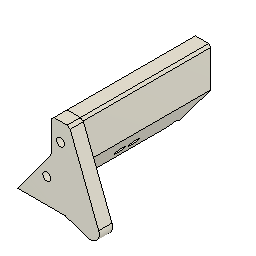
doctor-blade-coater (Autodesk Fusion 360 design; units mm, degrees)
Autodesk Fusion 360 part; units mm, degrees
note: some values were not read from the file. Set by a fixed rule: which sketch regions a step uses; the direction of a hole.
sketch "Blade Stock Layout and Angle setting" plane through (0, 0, 0) normal (0, 0, 1) x (1, 0, 0) in component "Blade"
  line L0 (0, 1.52) -> (0.9475, 3.3067)
  line L1 (0, 1.52) -> (1.43, 2.95)
  line L2 (0.9475, 3.3067) -> (1.43, 2.95) construction
  line L3 (1.43, 2.95) -> (11.5347, 16.621)
  line L4 (11.5347, 16.621) -> (11.0522, 16.9777)
  line L5 (11.0522, 16.9777) -> (0.9475, 3.3067)
  line L6 (0, 1.52) -> (0, 0) construction
  line L7 (0, 0) -> (17.3611, 0) construction
  dimension "d6" = 1.52
  dimension "d8" = 0.6
  dimension "d9" = 2
  dimension "d10" = 19
  dimension "d11" = 45
  constraint perpendicular L2 L3
  constraint parallel L2 L4
  constraint parallel L3 L5
  constraint equal L0 L1
  constraint vertical L6.end L0.start
  constraint coincident L6.end L7.start
  constraint perpendicular L6 L7
  measures "d6" distance of L0.start L6.end
  measures "d8" distance of L3.end L4.end
  measures "d9" distance of L0.start L2
  measures "d10" distance of L0.start L4
  measures "d11" angle of L1 L7
extrude "Blade Stock" add sketch "Blade Stock Layout and Angle setting" along normal mid plane 60 makes body 1 in component "Blade"
sketch "Blade profile" plane through (-0.9678, 0.7153, 0) normal (-0.804176, 0.594391, 0) x (0, 0, 1) in component "Blade"
  line L0 (-30, 20.2223) -> (-30, 3.2223)
  line L1 (-30, 3.2223) -> (30, 3.2223) construction
  line L2 (30, 3.2223) -> (30, 20.2223)
  line L3 (30, 20.2223) -> (-30, 20.2223)
  line L4 (0, 20.2223) -> (0, 3.2223) construction
  line L5 (30, 1.2223) -> (15, 20.2223)
  circle A0 centre (3.2, 17.8223) radius 1.7
  line L6 (1.5, 17.8223) -> (1.5, 20.2223)
  line L7 (4.9, 17.8223) -> (4.9, 20.2223)
  line L8 (3.2, 20.2223) -> (3.2, 16.1223) construction
  circle A1 centre (-3.2, 17.8223) radius 1.7
  line L9 (-1.5, 17.8223) -> (-1.5, 20.2223)
  line L10 (-4.9, 17.8223) -> (-4.9, 20.2223)
  line L11 (-30, 1.2223) -> (-15, 20.2223)
  line L12 (30, 1.2223) -> (30, 3.2223)
  line L13 (-30, 1.2223) -> (-30, 3.2223)
  point P0 (30, 1.2223)
  dimension "d20" = 15
  dimension "d21" = 3.4
  dimension "d22" = 1.5
  dimension "d23" = 4.1
  constraint midpoint L3 L4.start
  constraint midpoint L1 L4.end
  constraint coincident P0 L5.start
  constraint coincident L3 L5.end
  constraint coincident A0 L6.start
  constraint coincident L3 L6.end
  constraint tangent A0 L6
  constraint vertical L6
  constraint coincident A0 L7.start
  constraint coincident L3 L7.end
  constraint tangent A0 L7
  constraint vertical L7
  constraint coincident L3 L8.start
  constraint coincident A0 L8.end
  constraint perpendicular L3 L8
  constraint coincident A0.centre L8
  constraint symmetric L4 P0 L11.start
  constraint symmetric L4 L5.end L11.end
  constraint symmetric L4 A0 A1
  constraint symmetric L4 L6.start L9.start
  constraint symmetric L4 L6.end L9.end
  constraint symmetric L4 L7.start L10.start
  constraint symmetric L4 L7.end L10.end
  constraint coincident L1.end L2.start
  constraint symmetric L4 L1.end L0.end
  measures "d20" distance of L4 L5.end
  measures "d21" diameter of A0
  measures "d22" distance of L4 L6.end
  measures "d23" distance of L8.start L8.end
extrude "Blaade profile" cut sketch "Blade profile" against normal through all bodies 1 in component "Blade"
sketch "Blade Holder Stock Layout" plane through (0, 0, 0) normal (0, 0, 1) x (1, 0, 0) in component "Blade Holder"
  line L0 (0.9475, 3.3067) -> (0, 1.52)
  line L1 (0, 1.52) -> (1.43, 2.95)
  line L2 (1.43, 2.95) -> (11.5347, 16.621)
  line L3 (11.5347, 16.621) -> (11.0522, 16.9777)
  line L4 (11.0522, 16.9777) -> (0.9475, 3.3067)
  line L5 (1.2783, 3.7542) -> (11.9725, 3.7542)
  line L6 (11.9725, 3.7542) -> (25.4679, 22.0127)
  line L7 (11.5347, 16.621) -> (17.4679, 24.6483)
  line L8 (17.4679, 24.6483) -> (17.4679, 39.6483)
  line L9 (17.4679, 39.6483) -> (25.4679, 39.6483)
  line L10 (25.4679, 39.6483) -> (25.4679, 22.0127)
  line L11 (17.4679, 24.6483) -> (25.4679, 24.6483) construction
  line L12 (17.4679, 24.6483) -> (23.9013, 19.8932) construction
  line L13 (11.5347, 16.621) -> (1.43, 2.95)
  point P0 (2.0244, 3.7542)
  dimension "d30" = 8
  dimension "d31" = 15
  dimension "d32" = 10
  dimension "d40" = 1
  constraint horizontal L5
  constraint parallel L2 L6
  constraint vertical L8
  constraint perpendicular L8 L9
  constraint vertical L10
  constraint coincident L10 L11.end
  constraint perpendicular L10 L11
  constraint coincident L6 L12.end
  constraint perpendicular L6 L12
  constraint equal L11 L12
  constraint coincident L4 L5.start
  constraint coincident L2.end L3.start
  constraint parallel L6 L7
  constraint coincident L13 P0
  constraint coincident L5 P0
  measures "d30" distance of L2 L6
  measures "d31" distance of L7.end L8.end
  measures "d32" distance of L3.end L7.end
  measures "d40" distance of L1.end P0
extrude "Blade Holder Stock" add sketch "Blade Holder Stock Layout" along normal mid plane 58 separate body contours L2 L5 L6 L7 L8 L9 L10 L13 makes body 2 in component "Blade Holder"
sketch "Blade holder lateral stops layout" plane through (-0.4853, 0.3587, 0) normal (-0.804176, 0.594391, 0) x (0, 0, 1) in component "Blade Holder"
  line L0 (-29, 4.2223) -> (29, 4.2223)
  line L1 (29, 4.2223) -> (29, 30.2043)
  line L2 (-29, 30.2043) -> (-29, 4.2223)
  line L3 (28.4211, 3.2223) -> (15, 20.2223)
  line L4 (14.9301, 20.795) -> (28.0138, 4.2223)
  line L5 (0, 1.4073) -> (0, 18.094)
  line L6 (-14.9301, 20.795) -> (-28.0138, 4.2223)
  circle A0 centre (25.5, 9.8272) radius 1.5 construction
  line L7 (25.5, 9.8272) -> (27, 9.8272) construction
  line L8 (27, 9.8272) -> (29, 9.8272) construction
  line L9 (29, 30.2043) -> (-29, 30.2043)
  line L10 (4.9, 20.2223) -> (15, 20.2223)
  line L11 (-1.5, 20.2223) -> (1.5, 20.2223) construction
  line L12 (-15, 20.2223) -> (-4.9, 20.2223)
  line L13 (4.9, 20.2223) -> (1.5, 20.2223) construction
  line L14 (-1.5, 20.2223) -> (-4.9, 20.2223) construction
  line L15 (15, 20.2223) -> (15.3822, 20.2223)
  line L16 (-15, 20.2223) -> (-15.3822, 20.2223)
  line L17 (18.5401, 16.2223) -> (19.7174, 17.1518)
  line L18 (19.7174, 17.1518) -> (16.1091, 21.7223)
  line L19 (16.1091, 21.7223) -> (0, 21.7223)
  line L20 (0, 21.7223) -> (0, 20.2223) construction
  line L21 (-16.1091, 21.7223) -> (0, 21.7223)
  line L22 (-19.7174, 17.1518) -> (-16.1091, 21.7223)
  line L23 (-18.5401, 16.2223) -> (-19.7174, 17.1518)
  line L24 (9.95, 20.2223) -> (9.95, 21.7223)
  line L25 (-9.95, 20.2223) -> (-9.95, 21.7223)
  dimension "d42" = 0.3
  dimension "d93" = 3
  dimension "d94" = 2
  dimension "d95" = 1.5
  dimension "d97" = 4
  constraint coincident L0 L4.end
  constraint parallel L3 L4
  constraint symmetric L4.start L5 L6.start
  constraint symmetric L4.end L5 L6.end
  constraint coincident L4 L17.start
  constraint tangent L4 A0
  constraint coincident A0.centre L7.start
  constraint coincident A0 L7.end
  constraint horizontal L7
  constraint coincident L1 L8.end
  constraint perpendicular L1 L8
  constraint coincident L10.start L13.start
  constraint coincident L11.end L13.end
  constraint coincident L11.start L14.start
  constraint coincident L12.end L14.end
  constraint coincident L3.end L10.end
  constraint coincident L4 L15.end
  constraint parallel L10 L15
  constraint coincident L12.start L16.start
  constraint coincident L6 L16.end
  constraint parallel L12 L16
  constraint perpendicular L4 L17
  constraint perpendicular L17 L18
  constraint midpoint L11 L20.end
  constraint vertical L20
  constraint equal L17 L20
  constraint symmetric L5 L17.start L23.start
  constraint symmetric L5 L17.end L22.start
  constraint symmetric L5 L18.end L21.start
  constraint symmetric L5 L19.end L20.start
  constraint midpoint L10 L24.start
  constraint coincident L19 L24.end
  constraint perpendicular L19 L24
  constraint symmetric L5 L24.start L25.start
  constraint symmetric L5 L24.end L25.end
  measures "d42" distance of L3 L4
  measures "d93" diameter of A0
  measures "d94" distance of L7.end L8.end
  measures "d95" distance of L10 L19
  measures "d97" vertical distance of L17.start L3.end
extrude "Extrude3" add sketch "Blade holder lateral stops layout" along normal up to surface (0.6 mm away) contours L6 L12 L16 L21 L22 L23 L25 | L4 L10 L15 L17 L18 L19 L24 bodies 2 in component "Blade Holder"
sketch "Blade hole layout in holder" plane through (-0.4853, 0.3587, 0) normal (-0.804176, 0.594391, 0) x (0, 0, 1) in component "Blade Holder"
  line L0 (-29, 4.2223) -> (29, 4.2223)
  arc A0 (-4.9, 17.8223) -> (-1.5, 17.8223) centre (-3.2, 17.8223) ccw
  arc A1 (1.5, 17.8223) -> (4.9, 17.8223) centre (3.2, 17.8223) ccw
  line L1 (-29, 30.2043) -> (-29, 4.2223)
  circle A2 centre (25.5, 9.8272) radius 1.5 construction
  line L2 (0, 1.4073) -> (0, 18.094)
  circle A3 centre (-25.5, 9.8272) radius 1.5 construction
  line L3 (29, 4.2223) -> (29, 30.2043)
  line L4 (29, 30.2043) -> (-29, 30.2043)
  line L5 (15.3822, 20.2223) -> (9.95, 20.2223)
  line L6 (9.95, 20.2223) -> (9.95, 21.7223)
  line L7 (9.95, 21.7223) -> (16.1091, 21.7223)
  line L8 (16.1091, 21.7223) -> (19.7174, 17.1518)
  line L9 (-19.7174, 17.1518) -> (-16.1091, 21.7223)
  line L10 (-16.1091, 21.7223) -> (-9.95, 21.7223)
  line L11 (-9.95, 21.7223) -> (-9.95, 20.2223)
  line L12 (-9.95, 20.2223) -> (-15.3822, 20.2223)
  line L13 (-15.3822, 20.2223) -> (-18.5401, 16.2223)
  line L14 (-18.5401, 16.2223) -> (-19.7174, 17.1518)
  line L15 (19.7174, 17.1518) -> (18.5401, 16.2223)
  line L16 (18.5401, 16.2223) -> (15.3822, 20.2223)
  constraint symmetric A2 L2 A3
hole "Hole1" at (10.1081, 14.691, -3.2) at (10.1081, 14.691, 3.2) at (5.3559, 8.2615, 25.5) at (5.3559, 8.2615, -25.5) direction (0.804176, -0.594391, 0) diameter 4.35 end through all bodies 2 in component "Blade Holder"
sketch "Support Arm Stock Layout" plane through (0, 0, 29) normal (0, 0, 1) x (1, 0, 0) in component "Support Arm"
  line L0 (17.4679, 24.6483) -> (2.0244, 3.7542)
  line L1 (2.0244, 3.7542) -> (11.9725, 3.7542)
  line L2 (11.9725, 3.7542) -> (25.4679, 22.0127)
  line L3 (25.4679, 22.0127) -> (25.4679, 39.6483)
  line L4 (25.4679, 39.6483) -> (17.4679, 39.6483)
  line L5 (17.4679, 39.6483) -> (17.4679, 24.6483)
  line L6 (0, 0) -> (35, 0) construction
  line L7 (38.7295, 5.4461) -> (25.4679, 39.6483)
  circle A0 centre (35, 4) radius 4
  line L8 (23.4862, 3.7542) -> (33.691, 0.2202)
  line L9 (11.9725, 3.7542) -> (35, 3.7542) construction
  line L10 (35, 3.7542) -> (35, 4) construction
  line L11 (23.4862, 3.7542) -> (11.9725, 3.7542)
  line L12 (17.4679, 32.1483) -> (25.4679, 30.8305) construction
  line L13 (12.0583, 17.3295) -> (18.4917, 12.5743) construction
  line L14 (4.0631, 6.5124) -> (6.6487, 10.0106)
  line L15 (6.6487, 10.0106) -> (17.4679, 24.6483)
  point P0 (21.4679, 31.4894)
  point P1 (15.275, 14.9519)
  dimension "d58" = 8
  dimension "d61" = 35
  constraint coincident L6.start origin
  constraint horizontal L6
  constraint coincident L3.end L4.start
  constraint coincident L7.start A0
  constraint tangent L7 A0
  constraint tangent L6 A0
  constraint coincident A0 L8.end
  constraint tangent A0 L8
  constraint coincident L6.end A0
  constraint coincident L1.end L2.start
  constraint coincident A0.centre L10.end
  constraint vertical L10
  constraint horizontal L9
  constraint midpoint L8.start L9
  constraint midpoint L5 L12.start
  constraint midpoint L3 L12.end
  constraint coincident L2 L13.end
  constraint perpendicular L2 L13
  constraint midpoint L12 P0
  constraint midpoint L13 P1
  constraint coincident L0 L13.start
  constraint coincident L14.end L15.start
  constraint coincident L0.start L5.end
  constraint midpoint L13.start L15
  measures "d58" diameter of A0
  measures "d61" distance of L6.start L6.end
extrude "Support Arm Stock" add sketch "Support Arm Stock Layout" along normal blind 6 separate body makes body 3 in component "Support Arm"
hole "Hole1'" at (15.275, 14.9519, 29) at (21.4679, 31.4894, 29) direction (0, 0, 1) diameter 3.6 end through all bodies 3 in component "Support Arm"
sketch "Support arm hole layout in holder" plane through (0, 0, 29) normal (0, 0, 1) x (1, 0, 0) in component "Blade Holder"
  line L0 (17.4679, 24.6483) -> (2.0244, 3.7542)
  line L1 (2.0244, 3.7542) -> (11.9725, 3.7542)
  line L2 (11.9725, 3.7542) -> (25.4679, 22.0127)
  line L3 (25.4679, 22.0127) -> (25.4679, 39.6483)
  line L4 (25.4679, 39.6483) -> (17.4679, 39.6483)
  line L5 (17.4679, 39.6483) -> (17.4679, 24.6483)
  circle A0 centre (21.4679, 31.4894) radius 1.8
  circle A1 centre (15.275, 14.9519) radius 1.8
hole "support arm holes in holder" at (21.4679, 31.4894, 29) at (15.275, 14.9519, 29) direction (0, 0, -1) diameter 4.35 depth 8 tip angle 180 bodies 2 in component "Blade Holder"
chamfer "Support Arm chamfers" distance 1 angle 45 3 edges at (17.4679, 39.6483, 32) (25.4679, 39.6483, 32) (17.4679, 24.6483, 32) on bodies 3 in component "Support Arm"
chamfer "Blade Holder Chamfers" distance 1 angle 45 3 edges at (17.4679, 39.6483, 0) (17.4679, 24.6483, 0) (25.4679, 39.6483, 0) on bodies 2 in component "Blade Holder"
fillet "lateral Stops Fillets" radius 0.75 4 edges at (9.4683, 14.3301, 19.7174) (8.9159, 13.5826, 18.5401) (11.2934, 16.7993, 9.95) (12.185, 18.0056, 9.95) on bodies 2 in component "Blade Holder"
fillet "lateral Stops Fillets" radius 0.75 4 edges at (8.9159, 13.5826, -18.5401) (11.2934, 16.7993, -9.95) (12.185, 18.0056, -9.95) (9.4683, 14.3301, -19.7174) on bodies 2 in component "Blade Holder"
component "Blade" placed x (1, 0, 0) y (0, 1, 0) z (0, 0, 1) at (0, 0, 0)
component "Blade Holder" placed x (1, 0, 0) y (0, 1, 0) z (0, 0, 1) at (0, 0, 0)
component "Support Arm" placed x (1, 0, 0) y (0, 1, 0) z (0, 0, 1) at (0, 0, 0)
equation "blade_thickness = 0.6 mm"
equation "blade_width = 19 mm"
equation "edge_width = 2 mm"
equation "blade_height = 1.52 mm" comment "INPUT: Height of the blade above the reference surface"
equation "d6 = blade_height"
equation "d8 = blade_thickness"
equation "d9 = edge_width"
equation "d10 = blade_width"
equation "d11 = blade_angle"
equation "blade_angle = 45 deg" comment "Angle between the blade and the reference surface"
equation "edge_length = 60 mm"
equation "d14 = edge_length"
equation "blade_body_length = 30 mm"
equation "blade_cutout_depth = 4.1 mm"
equation "blade_cutout_width = 3.4 mm"
equation "blade_tab_width = 3 mm"
equation "d20 = blade_body_length / 2"
equation "d21 = blade_cutout_width"
equation "d22 = blade_tab_width / 2"
equation "d23 = blade_cutout_depth"
equation "handle_thickness = 8 mm"
equation "edge_holder_offset = 1 mm" comment "Extent of blade edge beyond the holder"
equation "handle_height = 15 mm"
equation "edge_handle_offset = 10 mm" comment "Distance between the top of the blade and the start of the handle"
equation "d30 = handle_thickness"
equation "d31 = handle_height"
equation "d32 = edge_handle_offset"
equation "blade_holder_length = 58 mm"
equation "d34 = blade_holder_length"
equation "blade_width_offset = 0.3 mm"
equation "d40 = edge_holder_offset"
equation "d42 = blade_width_offset"
equation "M3_threaded_insert_diameter = 4.35 mm"
equation "M3_threaded_insert_depth = 8 mm"
equation "d48 = M3_threaded_insert_diameter"
equation "support_arm_thickness = 6 mm"
equation "support_arm_edge_separation = 35 mm" comment "Horizontal distance between the edge and the point of contact of the support arm with the reference surface"
equation "support_arm_radius = 4 mm" comment "Radius of the point of comtact of the support arm with the reference surface"
equation "d58 = support_arm_radius * 2"
equation "d61 = support_arm_edge_separation"
equation "d62 = support_arm_thickness"
equation "M3_clearance_diameter = 3.6 mm"
equation "d66 = M3_clearance_diameter"
equation "d68 = M3_threaded_insert_depth"
equation "d69 = M3_threaded_insert_diameter"
equation "bladeClampWidthOffsets = 1 mm"
equation "blade_clamp_height_offset = 1 mm"
equation "blade_clamp_height_extent = 2 mm" comment "Vertical Extent of Clamp above top edge of blade"
equation "clamp_thickness = 8 mm"
equation "clamp_chamfer = 5 mm"
equation "d94 = side_bolt_offset"
equation "d95 = lateral_stop_width"
equation "d97 = lateral_stop_vertical_extent"
equation "lateral_stop_width = 1.5 mm"
equation "lateral_stop_vertical_extent = 4 mm"
equation "side_bolt_offset = 2 mm"
